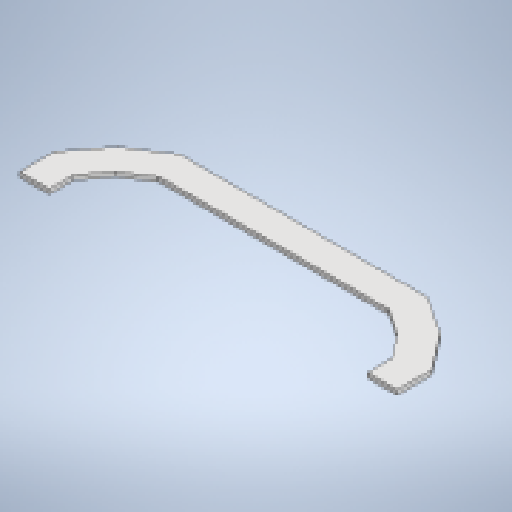
# Autodesk Inventor part: przód
Saved by Autodesk Inventor 2023 (Build 270158000, 158)
## iProperties
Created: 2024-03-30
Part Number: przód
Material: Ogólny
Document SubType Name: Modeling
Designer: Kamil
Density: 1 g/cm^3
Appearance: Domyślna
Author: Kamil
Autodesk Inventor part; units mm, degrees
ref_plane "YZ Plane" through (0, 0, 0) normal (1, 0, 0) x (0, 1, 0)
ref_plane "XZ Plane" through (0, 0, 0) normal (0, 1, 0) x (-1, 0, 0)
ref_plane "XY Plane" through (0, 0, 0) normal (0, 0, 1) x (1, 0, 0)
sketch "Szkic2" plane through (0, 0, 0) normal (0, 1, 0) x (-1, 0, 0)
  line L0 (47.5, 5) -> (-47.5, 5)
  line L1 (-47.5, 5) -> (-47.5, -5)
  line L2 (-47.5, -5) -> (47.5, -5)
  line L3 (47.5, -5) -> (47.5, 5)
  line L4 (47.5, 5) -> (-47.5, -5) construction
  line L5 (-47.5, 5) -> (47.5, -5) construction
  line L6 (0, 24) -> (0, -27)
  point P0 (0, 0)
  dimension "d10" = 10
  dimension "d11" = 95
  constraints: 14 end point, 2 midpoint, 2 parallel, 2 vertical, 1 horizontal, 1 perpendicular
  measures "d10" distance of L2.end L0.start
  measures "d11" distance of L1.end L2.end
extrude "Wyciągnięcie proste2" add sketch "Szkic2" along normal blind 1.6
sketch "Szkic3" plane through (0, 1.6, 0) normal (0, 1, 0) x (1, 0, 0)
  line L0 (-47.5, -5) -> (47.5, -5) projected
  line L1 (47.5, -5) -> (47.5, 5) projected
  line L2 (47.5, 5) -> (-47.5, 5) projected
  line L3 (-47.5, 5) -> (-47.5, -5) projected
  line L4 (52, -8.65) -> (49.4, -5.35) construction
  line L5 (59.75, -18.7) -> (57.1, -15.35) construction
  line L6 (41.3, -1.65) -> (38.65, 1.7) construction
  line L7 (58.425, -17.025) -> (50.7, -7) construction
  line L8 (39.975, 0.025) -> (50.7, -7) construction
  line L9 (58.425, -17.025) -> (58.425, -30) construction
  line L10 (38.5214, -5) -> (47.2545, -10.7203)
  line L11 (47.2545, -10.7203) -> (53.425, -18.728)
  line L12 (53.425, -18.728) -> (53.425, -27.025)
  line L13 (41.5049, 5) -> (54.1455, -3.2797)
  line L14 (54.1455, -3.2797) -> (63.425, -15.322)
  line L15 (63.425, -15.322) -> (63.425, -27.025)
  line L16 (63.425, -27.025) -> (53.425, -27.025)
  line L17 (0, -5) -> (0, 20.232)
  line L18 (-38.5214, -5) -> (-47.2545, -10.7203)
  line L19 (-47.2545, -10.7203) -> (-53.425, -18.728)
  line L20 (-53.425, -18.728) -> (-53.425, -27.025)
  line L21 (-41.5049, 5) -> (-54.1455, -3.2797)
  line L22 (-54.1455, -3.2797) -> (-63.425, -15.322)
  line L23 (-63.425, -15.322) -> (-63.425, -27.025)
  line L24 (-63.425, -27.025) -> (-53.425, -27.025)
  point P0 (0, 0)
  point P1 (-47.5, 1.0732)
  point P2 (47.5, 1.0732)
  dimension "d17" = 5
  dimension "d18" = 5
  dimension "d19" = 10
  constraints: 42 end point, 8 symmetric about line, 5 midpoint, 2 point on line, 2 vertical, 1 horizontal, 10 other
  measures "d17" distance between parallel lines of L7 L11
  measures "d18" distance between parallel lines of L7 L14
  measures "d19" distance from line of L16 L7.start
extrude "Wyciągnięcie proste3" add sketch "Szkic3" against normal up to surface (1.6 mm away) contours L0 L18 L19 L20 L24 L23 L22 L21 L3 | L0 L1 L13 L14 L15 L16 L12 L11 L10
extrude "Wyciągnięcie proste4" cut sketch "Szkic3" against normal through all contours L3 L2 L21 | L2 L1 L13
sketch "Szkic4" plane through (0, 1.6, 0) normal (0, 1, 0) x (1, 0, 0)
  line L0 (-41.5049, 5) -> (-54.1455, -3.2797) projected
  line L1 (-54.1455, -3.2797) -> (-63.425, -15.322) projected
  line L2 (-63.425, -15.322) -> (-63.425, -27.025) projected
  line L3 (-63.425, -27.025) -> (-53.425, -27.025) projected
  line L4 (-53.425, -27.025) -> (-53.425, -18.728) projected
  line L5 (-53.425, -18.728) -> (-47.2545, -10.7203) projected
  line L6 (-47.2545, -10.7203) -> (-38.5214, -5) projected
  line L7 (-38.5214, -5) -> (38.5214, -5) projected
  line L8 (38.5214, -5) -> (47.2545, -10.7203) projected
  line L9 (47.2545, -10.7203) -> (53.425, -18.728) projected
  line L10 (53.425, -18.728) -> (53.425, -27.025) projected
  line L11 (53.425, -27.025) -> (63.425, -27.025) projected
  line L12 (63.425, -27.025) -> (63.425, -15.322) projected
  line L13 (63.425, -15.322) -> (54.1455, -3.2797) projected
  line L14 (54.1455, -3.2797) -> (41.5049, 5) projected
  line L15 (41.5049, 5) -> (-41.5049, 5) projected
  line L16 (41.5049, 5) -> (35.3982, 9)
  line L17 (35.3982, 9) -> (-35.3982, 9)
  line L18 (-35.3982, 9) -> (-41.5049, 5)
  point P0 (0, 0)
  dimension "d24" = 4
  constraints: 6 end point, 2 collinear, 1 horizontal
  measures "d24" distance between parallel lines of L17 L15
extrude "Wyciągnięcie proste5" add sketch "Szkic4" against normal up to surface (1.6 mm away) contours L18 L17 L16 L15
sketch "Szkic5" plane through (0, 1.6, 0) normal (0, 1, 0) x (1, 0, 0)
  line L0 (-35.3982, 9) -> (-54.1455, -3.2797) projected
  line L1 (-54.1455, -3.2797) -> (-63.425, -15.322) projected
  line L2 (-63.425, -15.322) -> (-63.425, -27.025) projected
  line L3 (-63.425, -27.025) -> (-53.425, -27.025) projected
  line L4 (-53.425, -27.025) -> (-53.425, -18.728) projected
  line L5 (-53.425, -18.728) -> (-47.2545, -10.7203) projected
  line L6 (-47.2545, -10.7203) -> (-38.5214, -5) projected
  line L7 (-38.5214, -5) -> (38.5214, -5) projected
  line L8 (38.5214, -5) -> (47.2545, -10.7203) projected
  line L9 (47.2545, -10.7203) -> (53.425, -18.728) projected
  line L10 (53.425, -18.728) -> (53.425, -27.025) projected
  line L11 (53.425, -27.025) -> (63.425, -27.025) projected
  line L12 (63.425, -27.025) -> (63.425, -15.322) projected
  line L13 (63.425, -15.322) -> (54.1455, -3.2797) projected
  line L14 (54.1455, -3.2797) -> (35.3982, 9) projected
  line L15 (35.3982, 9) -> (-35.3982, 9) projected
  line L16 (-15, -5) -> (15, -5)
  line L17 (15, -5) -> (15, -15)
  line L18 (15, -15) -> (-15, -15)
  line L19 (-15, -15) -> (-15, -5)
  point P0 (0, 0)
  point P1 (0, -5)
  point P2 (0, 0)
  point P3 (0, -5)
  point P4 (0, -5)
  dimension "d27" = 30
  dimension "d28" = 10
  constraints: 8 end point, 3 coincident, 2 midpoint, 2 parallel, 1 horizontal, 1 perpendicular, 1 vertical alignment
  measures "d27" distance of L17.end L18.end
  measures "d28" distance of L16.end L17.end
extrude "Wyciągnięcie proste6" add sketch "Szkic5" against normal up to surface (1.6 mm away) contours L7 L17 L18 L19
fillet "Zaokrąglenie1" radius 10 12 edges at (-63.425, 0.8, 15.322) (-54.1455, 0.8, 3.2797) (-35.3982, 0.8, -9) (35.3982, 0.8, -9) (54.1455, 0.8, 3.2797) (63.425, 0.8, 15.322) (-53.425, 0.8, 18.728) (-47.2545, 0.8, 10.7203) (-38.5214, 0.8, 5) (38.5214, 0.8, 5) (47.2545, 0.8, 10.7203) (53.425, 0.8, 18.728)
fillet "Zaokrąglenie2" radius 4 2 edges at (-15, 0.8, 5) (15, 0.8, 5)
fillet "Zaokrąglenie3" radius 2 2 edges at (15, 0.8, 15) (-15, 0.8, 15)
sketch "Szkic6" plane through (0, 1.6, 0) normal (0, 1, 0) x (1, 0, 0)
  line L0 (32.4146, 9) -> (-32.4146, 9) projected
  line L1 (-5, 9) -> (5, 9)
  line L2 (5, 9) -> (5, 29)
  line L3 (5, 29) -> (-5, 29)
  line L4 (-5, 29) -> (-5, 9)
  point P0 (0, 0)
  point P1 (0, 9)
  point P2 (0, 9)
  dimension "d34" = 10
  dimension "d35" = 20
  constraints: 8 end point, 2 midpoint, 2 parallel, 1 coincident, 1 horizontal, 1 perpendicular, 1 vertical alignment
  measures "d34" distance of L3.end L2.end
  measures "d35" distance of L2.end L1.end
extrude "Wyciągnięcie proste7" add sketch "Szkic6" against normal up to surface (1.6 mm away)
fillet "Zaokrąglenie4" radius 4 2 edges at (5, 0.8, -9) (-5, 0.8, -9)
fillet "Zaokrąglenie5" radius 1 2 edges at (5, 0.8, -29) (-5, 0.8, -29)
fillet "Zaokrąglenie6" radius 1 4 edges at (-63.425, 0.8, 27.025) (-53.425, 0.8, 27.025) (53.425, 0.8, 27.025) (63.425, 0.8, 27.025)
